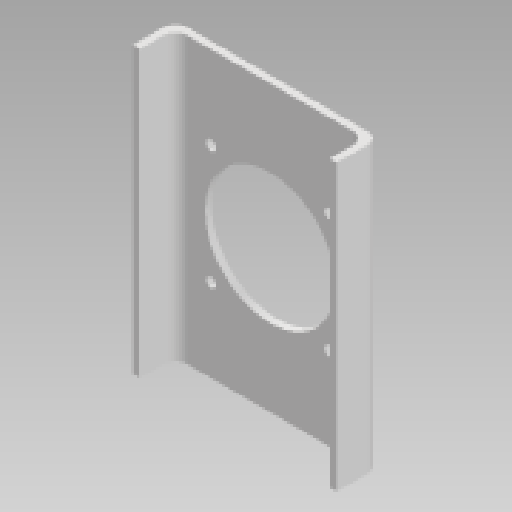
# Autodesk Inventor part: FanHolder
Saved by Autodesk Inventor 2026.1 (Build 301233000, 233)
## iProperties
Created: 2026-02-27
Part Number: FanHolder
Material: Generic
Document SubType Name: Modeling
Designer: aleja
Density: 1 g/cm^3
Appearance: Default
Author: aleja
Autodesk Inventor part; units mm, degrees
ref_plane "YZ Plane" through (0, 0, 0) normal (1, 0, 0) x (0, 1, 0)
ref_plane "XZ Plane" through (0, 0, 0) normal (0, 1, 0) x (-1, 0, 0)
ref_plane "XY Plane" through (0, 0, 0) normal (0, 0, 1) x (1, 0, 0)
sketch "Sketch1" plane through (0, 0, 0) normal (0, 0, 1) x (1, 0, 0)
  line L0 (0, 0) -> (40, 0)
  line L1 (0, 0) -> (0, -20) construction
  line L2 (40, 0) -> (40, -15.5)
  line L3 (0, 0) -> (40, 0)
  line L4 (40, 0) -> (40, 3)
  line L5 (40, 3) -> (0, 3)
  line L6 (0, 3) -> (0, 0)
  line L7 (40, 3) -> (43, 3)
  line L8 (43, 3) -> (43, -15.5)
  line L9 (43, -15.5) -> (40, -15.5)
  line L10 (40, -15.5) -> (40, 3)
  line L11 (0, 0) -> (-40, 0)
  line L12 (-40, 0) -> (-40, -15.5)
  line L13 (-40, 3) -> (0, 3)
  line L14 (-40, 3) -> (-43, 3)
  line L15 (-43, 3) -> (-43, -15.5)
  line L16 (-43, -15.5) -> (-40, -15.5)
  point P0 (41.5, -15.5)
  dimension "d0" = 40
  dimension "d1" = 20
  dimension "d3" = 3
  dimension "d4" = 3
  dimension "d17" = 15.5
  constraints: 34 end point, 6 symmetric about line, 4 parallel, 3 horizontal, 2 perpendicular, 2 vertical, 1 midpoint
  measures "d0" distance of L0.start L0.end
  measures "d1" distance of L0.start L1.end
  measures "d3" distance of L4.end L3.end
  measures "d4" distance of L8.end L9.end
  measures "d17" distance from line of L0 point (41.5, -15.5)
extrude "Extrusion1" add sketch "Sketch1" along normal blind 120
sketch "Sketch2" plane through (-43, 3, 0) normal (0, 1, 0) x (1, 0, 0)
  line L0 (86, 0) -> (86, -120) projected
  line L1 (86, -60) -> (0, -60) construction
  line L2 (0, 0) -> (0, -120) projected
  line L3 (68, -35) -> (18, -35) construction
  line L4 (18, -35) -> (18, -85) construction
  line L5 (18, -85) -> (68, -85) construction
  line L6 (68, -85) -> (68, -35) construction
  line L7 (68, -35) -> (18, -85) construction
  line L8 (18, -35) -> (68, -85) construction
  circle A0 centre (68, -85) radius 2.15
  circle A1 centre (18, -85) radius 2.15
  circle A2 centre (68, -35) radius 2.15
  circle A3 centre (18, -35) radius 2.15
  circle A4 centre (43, -60) radius 27.5
  point P0 (43, 0)
  dimension "d7" = 50
  dimension "d8" = 50
  dimension "d9" = 4.3
  dimension "d10" = 4.3
  dimension "d11" = 4.3
  dimension "d12" = 4.3
  dimension "d15" = 55
  constraints: 14 end point, 5 centre point, 5 coincident, 5 midpoint, 2 parallel, 1 horizontal, 1 perpendicular
  measures "d7" distance of L5.end L4.end
  measures "d8" distance of L4.end L3.end
  measures "d9" diameter of A0
  measures "d10" diameter of A1
  measures "d11" diameter of A2
  measures "d12" diameter of A3
  measures "d15" diameter of A4
extrude "Extrusion2" cut sketch "Sketch2" against normal through all
fillet "Fillet1" radius 5 4 edges at (40, 0, 60) (43, 3, 60) (-40, 0, 60) (-43, 3, 60)
body "Solid1"
